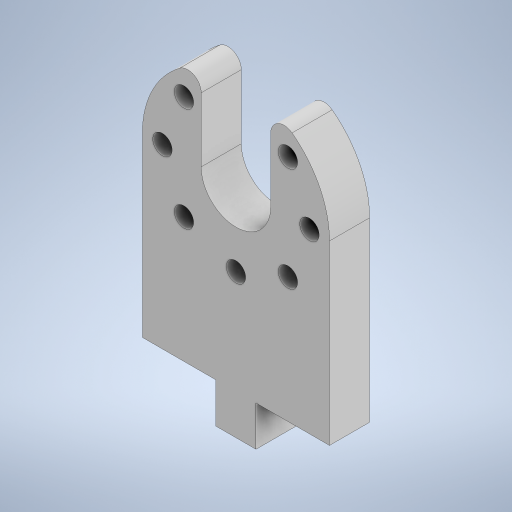
# Autodesk Inventor part: thighs_waist_connect
Saved by Autodesk Inventor 2024 (Build 280153000, 153)
## iProperties
Created: 2024-09-18
Part Number: thighs_waist_connect
Material: 일반
Document SubType Name: Modeling
Designer: Eungang
Density: 1 g/cm^3
Appearance: 기본값
Author: Eungang
Autodesk Inventor part; units mm, degrees
ref_plane "YZ Plane" through (0, 0, 0) normal (1, 0, 0) x (0, 1, 0)
ref_plane "XZ Plane" through (0, 0, 0) normal (0, 1, 0) x (-1, 0, 0)
ref_plane "XY Plane" through (0, 0, 0) normal (0, 0, 1) x (1, 0, 0)
sketch "스케치1" plane through (0, 0, 0) normal (0, 0, 1) x (1, 0, 0)
  circle A0 centre (0, 0) radius 14 projected
  circle A1 centre (-7.7782, 7.7782) radius 1.45
  circle A2 centre (-11, 0) radius 1.45
  circle A3 centre (-7.7782, -7.7782) radius 1.45
  circle A4 centre (0, -11) radius 1.45
  circle A5 centre (7.7782, -7.7782) radius 1.45
  circle A6 centre (11, 0) radius 1.45
  circle A7 centre (7.7782, 7.7782) radius 1.45
  circle A8 centre (0, 11) radius 1.45
  arc A9 (-5.2, 0) -> (5.2, 0) centre (0, 0) ccw
  line L0 (-5.2, 0) -> (5.2, 0)
  line L1 (5.2, 0) -> (5.2, 9.6)
  line L2 (-5.2, 9.6) -> (-5.2, 0)
  arc A10 (-8.4, 11.2) -> (8.4, 11.2) centre (0, 0) ccw
  arc A11 (-5.2, 9.6) -> (-8.4, 11.2) centre (-7.2, 9.6) ccw
  arc A12 (8.4, 11.2) -> (5.2, 9.6) centre (7.2, 9.6) ccw
  line L3 (22.8, -32.5) -> (-127.2, -32.5) projected
  line L4 (-127.2, -32.5) -> (-127.2, -26.5) projected
  line L5 (22.8, -26.5) -> (-127.2, -26.5) projected
  line L6 (22.8, -32.5) -> (22.8, -26.5) projected
  line L7 (14, 0) -> (-14, 0)
  line L8 (-14, 0) -> (-14, -26.5)
  line L9 (-14, -26.5) -> (14, -26.5)
  line L10 (14, -26.5) -> (14, 0)
  point P0 (5.2, 12.9985)
  point P1 (-5.2, 12.9985)
  point P2 (-8.4, 11.2)
  point P3 (8.4, 11.2)
  point P4 (14, -26.5)
  point P5 (-14, 0)
  dimension "d3" = 360
  dimension "d6" = 2
  constraints: 14 end point, 12 centre point, 11 point on circle, 4 tangent, 3 parallel, 3 point on line, 2 horizontal, 2 perpendicular, 1 coincident, 1 equal radius, 17 other
  measures "d6" radius of A11
extrude "돌출1" add sketch "스케치1" along normal blind 6 contours L7 A6 L1 A12 A0 | L10 L5 L8 A0 | A0 L7 A2 A9 A6 | A0 A11 L2 L7 A2
sketch "스케치2" plane through (-14, -26.5, 0) normal (0, -1, 0) x (1, 0, 0)
  line L0 (0, 0) -> (28, 0) projected
  line L1 (28, 0) -> (28, 6) projected
  line L2 (0, 6) -> (28, 6) projected
  line L3 (0, 0) -> (0, 6) projected
  line L4 (14, 6) -> (14, 0)
  line L5 (0, 6) -> (28, 6) projected
  line L6 (14, 0) -> (17, 0)
  line L7 (17, 0) -> (17, 6)
  line L8 (17, 6) -> (14, 6)
  line L9 (14, 6) -> (14, 0)
  line L10 (14, 0) -> (11, 0)
  line L11 (11, 0) -> (11, 6)
  line L12 (11, 6) -> (14, 6)
  line L13 (14, 6) -> (14, 0)
  dimension "d9" = 3
  dimension "d10" = 3
  constraints: 18 end point, 4 parallel, 2 horizontal, 2 perpendicular, 2 point on line, 1 midpoint, 1 vertical
  measures "d9" distance of L8.end L7.end
  measures "d10" distance of L11.end L12.end
extrude "돌출2" add sketch "스케치2" along normal blind 6 contours L11 L2 L4 L0 | L4 L2 L7 L0
